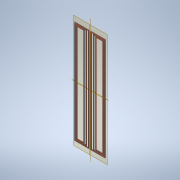
# Autodesk Inventor part: primary_coil
Saved by Autodesk Inventor 2020 (Build 240168000, 168)
## iProperties
Created: 2021-01-19
Part Number: primary_coil
Material: Generic
Document SubType Name: Modeling
Designer: phamv
Density: 1 g/cm^3
Appearance: Default
Author: phamv
Autodesk Inventor part; units mm, degrees
sketch "Sketch2" plane through (0, 0, 0) normal (0, 0, 1) x (1, 0, 0)
  line L0 (9, 500) -> (150, 500)
  line L1 (150, 500) -> (150, -500)
  line L2 (150, -500) -> (9, -500)
  line L3 (9, -500) -> (9, 500)
  line L4 (0, 0) -> (4.5229, 0) construction
  line L5 (-30, 0) -> (180, 0) construction
  line L6 (0, 700) -> (0, -700) construction
  line L7 (14, 495) -> (145, 495)
  line L8 (145, 495) -> (145, -495)
  line L9 (145, -495) -> (14, -495)
  line L10 (14, -495) -> (14, 495)
  line L11 (32, 490) -> (140, 490)
  line L12 (140, 490) -> (140, -490)
  line L13 (140, -490) -> (32, -490)
  line L14 (32, -490) -> (32, 490)
  line L15 (37, 485) -> (135, 485)
  line L16 (135, 485) -> (135, -485)
  line L17 (135, -485) -> (37, -485)
  line L18 (37, -485) -> (37, 485)
  line L19 (55, 480) -> (130, 480)
  line L20 (130, 480) -> (130, -480)
  line L21 (130, -480) -> (55, -480)
  line L22 (55, -480) -> (55, 480)
  line L23 (60, 475) -> (125, 475)
  line L24 (125, 475) -> (125, -475)
  line L25 (125, -475) -> (60, -475)
  line L26 (60, -475) -> (60, 475)
  point P0 (9, 0)
  point P1 (92.5, 475)
  dimension "d2" = 9
  dimension "d3" = 150
  dimension "d4" = 1000
  dimension "d5" = 5
  dimension "d6" = 5
  dimension "d7" = 5
  dimension "d8" = 5
  dimension "d9" = 18
  dimension "d10" = 5
  dimension "d11" = 5
  dimension "d12" = 5
  dimension "d13" = 5
  dimension "d14" = 5
  dimension "d15" = 5
  dimension "d16" = 5
  dimension "d17" = 18
  dimension "d18" = 5
  dimension "d19" = 5
  dimension "d20" = 5
  dimension "d21" = 5
  dimension "d22" = 5
  dimension "d23" = 5
  dimension "d24" = 5
  constraints: 50 end point, 12 parallel, 7 horizontal, 6 perpendicular, 2 midpoint, 1 coincident, 1 point on line
  measures "d2" distance between parallel lines of L3 L6
  measures "d3" distance between parallel lines of L1 L6
  measures "d4" distance between parallel lines of L2 L0
  measures "d5" distance between parallel lines of L3 L10
  measures "d6" distance between parallel lines of L7 L0
  measures "d7" distance between parallel lines of L2 L9
  measures "d8" distance between parallel lines of L1 L8
  measures "d9" distance between parallel lines of L10 L14
  measures "d10" distance between parallel lines of L8 L12
  measures "d11" distance between parallel lines of L11 L7
  measures "d12" distance between parallel lines of L9 L13
  measures "d13" distance between parallel lines of L18 L14
  measures "d14" distance between parallel lines of L11 L15
  measures "d15" distance between parallel lines of L12 L16
  measures "d16" distance between parallel lines of L13 L17
  measures "d17" distance between parallel lines of L22 L18
  measures "d18" distance between parallel lines of L15 L19
  measures "d19" distance between parallel lines of L16 L20
  measures "d20" distance between parallel lines of L17 L21
  measures "d21" distance between parallel lines of L22 L26
  measures "d22" distance between parallel lines of L19 L23
  measures "d23" distance between parallel lines of L20 L24
  measures "d24" distance between parallel lines of L21 L25
extrude "Extrusion1" add sketch "Sketch2" along normal blind 5
mirror "Mirror2" about plane through (0, 0, 0) normal (1, 0, 0) bodies 1 separate body
equation "\"d2\" = 0.5 * distance_between_wires"
equation "\"d3\" = 0.5 * track_width"
equation "\"d4\" = track_length"
equation "\"d5\" = wire_diameter"
equation "\"d6\" = wire_diameter"
equation "\"d7\" = wire_diameter"
equation "\"d8\" = wire_diameter"
equation "\"d9\" = distance_between_wires"
equation "\"d10\" = distance_between_wires_edge"
equation "\"d11\" = distance_between_wires_edge"
equation "\"d12\" = distance_between_wires_edge"
equation "\"d13\" = wire_diameter"
equation "\"d14\" = wire_diameter"
equation "\"d15\" = wire_diameter"
equation "\"d16\" = wire_diameter"
equation "\"d17\" = distance_between_wires"
equation "\"d18\" = distance_between_wires_edge"
equation "\"d19\" = distance_between_wires_edge"
equation "\"d20\" = distance_between_wires_edge"
equation "\"d21\" = wire_diameter"
equation "\"d22\" = wire_diameter"
equation "\"d23\" = wire_diameter"
equation "\"d24\" = wire_diameter"
equation "\"d25\" = wire_diameter"
equation "\"wire_diameter\" = 5"
equation "\"track_length\" = 1000"
equation "\"distance_between_wires\" = -1.2 * wire_diameter + 0.2 * parameter_6"
equation "\"distance_between_wires_edge\" = 5"
equation "\"track_width\" = 300"
equation "\"parameter_6\" = 120"
body "Solid1"
body "Solid2"
